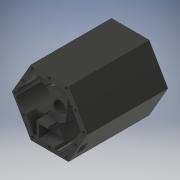
# Autodesk Inventor part: TA02
Saved by Autodesk Inventor 2017 (Build 210142000, 142)
## iProperties
Created: 2018-10-09
Part Number: TA02
Material: ABS Plastic
Document SubType Name: Modeling
Designer: Zach
Density: 1.06 g/cm^3
Appearance: Smooth - Black
Author: Zach
Autodesk Inventor part; units mm, degrees
ref_plane "YZ Plane" through (0, 0, 0) normal (1, 0, 0) x (0, 1, 0)
ref_plane "XZ Plane" through (0, 0, 0) normal (0, 1, 0) x (-1, 0, 0)
ref_plane "XY Plane" through (0, 0, 0) normal (0, 0, 1) x (1, 0, 0)
sketch "Sketch1" plane through (0, 0, 0) normal (0, 0, 1) x (1, 0, 0)
  circle A0 centre (0, 0) radius 56
  circle A1 centre (0, 0) radius 9.56
  circle A2 centre (-30, 0) radius 4
  line L0 (-39, 9) -> (-21, 9) construction
  line L1 (-21, 9) -> (-21, -9) construction
  line L2 (-21, -9) -> (-39, -9) construction
  line L3 (-39, -9) -> (-39, 9) construction
  circle A3 centre (-39, 9) radius 2
  circle A4 centre (-21, 9) radius 2
  circle A5 centre (-21, -9) radius 2
  circle A6 centre (-39, -9) radius 2
  circle A7 centre (15, 25.9808) radius 3.5
  line L4 (0, 0) -> (-30, 0) construction
  line L5 (0, 0) -> (15, 25.9808) construction
  line L6 (0, 0) -> (15, -25.9808) construction
  circle A8 centre (15, -25.9808) radius 3.5
  point P0 (-39, 0)
  point P1 (-30, 9)
  dimension "d0" = 112
  dimension "d1" = 19.12
  dimension "d2" = 8
  dimension "d3" = 30
  dimension "d4" = 18
  dimension "d5" = 18
  dimension "d6" = 4
  dimension "d7" = 4
  dimension "d8" = 4
  dimension "d9" = 4
  dimension "d10" = 7
  dimension "d11" = 30
  dimension "d12" = 120
  dimension "d13" = 30
  dimension "d14" = 7
  dimension "d15" = 120
  constraints: 14 end point, 9 centre point, 8 coincident, 2 horizontal, 2 horizontal alignment, 2 midpoint, 2 parallel, 1 perpendicular, 1 vertical alignment
  measures "d0" diameter of A0
  measures "d1" diameter of A1
  measures "d2" diameter of A2
  measures "d3" distance of L4.end point (0, 0)
  measures "d4" distance of L1.end L2.end
  measures "d5" distance of L0.end L1.end
  measures "d6" diameter of A3
  measures "d7" diameter of A4
  measures "d8" diameter of A5
  measures "d9" diameter of A6
  measures "d10" diameter of A7
  measures "d11" distance of L5.start L5.end
  measures "d12" angle of L5 L4
  measures "d13" distance of L5.start L6.end
  measures "d14" diameter of A8
  measures "d15" angle of L4 L6
extrude "Extrusion1" add sketch "Sketch1" along normal blind 5
sketch "Sketch2" plane through (0, 0, 5) normal (0, 0, 1) x (1, 0, 0)
  circle A0 centre (0, 0) radius 56 projected
  circle A1 centre (0, 0) radius 47
  dimension "d18" = 9
  constraints: 1 centre point, 1 coincident
  measures "d18" radial gap between concentric circles of A0 A1
extrude "Extrusion2" add sketch "Sketch2" along normal blind 115
sketch "Sketch3" plane through (0, 0, 5) normal (0, 0, 1) x (1, 0, 0)
  circle A0 centre (-30, 0) radius 4 projected
  circle A1 centre (0, 0) radius 9.56 projected
  circle A2 centre (15, 25.9808) radius 3.5 projected
  circle A3 centre (15, -25.9808) radius 3.5 projected
  circle A4 centre (-30, 0) radius 20
  line L0 (21.5753, 12.3695) -> (-0.0753, 24.8695)
  line L1 (-0.0753, 24.8695) -> (8.4247, 39.592)
  line L2 (8.4247, 39.592) -> (30.0753, 27.092)
  line L3 (30.0753, 27.092) -> (21.5753, 12.3695)
  line L4 (21.5753, 12.3695) -> (8.4247, 39.592) construction
  line L5 (-0.0753, 24.8695) -> (30.0753, 27.092) construction
  line L6 (0, 0) -> (-30, 0) construction
  line L7 (-0.0753, -24.8695) -> (21.5753, -12.3695)
  line L8 (21.5753, -12.3695) -> (30.0753, -27.092)
  line L9 (30.0753, -27.092) -> (8.4247, -39.592)
  line L10 (8.4247, -39.592) -> (-0.0753, -24.8695)
  circle A5 centre (0, 0) radius 47 projected
  dimension "d21" = 40
  dimension "d23" = 120
  dimension "d24" = 17
  dimension "d25" = 25
  dimension "d28" = 120
  constraints: 22 end point, 2 midpoint, 2 parallel, 1 centre point, 1 coincident, 1 horizontal, 1 perpendicular, 9 other
  measures "d21" diameter of A4
  measures "d23" angle of L6 L1
  measures "d24" distance of L0.end L1.end
  measures "d25" distance of L1.end L2.end
extrude "Extrusion3" add sketch "Sketch3" along normal blind 100 contours A4 A5 picked at (30.0502, 0)
sketch "Sketch6" plane through (-30, 0, 5) normal (0, 0, 1) x (0, 1, 0)
  circle A0 centre (0, 0) radius 4 projected
  circle A1 centre (0, 0) radius 16.5
  circle A2 centre (0, 0) radius 20 projected
  point P0 (0, -30)
  point P1 (-18.7483, -6.9642)
  dimension "d46" = 33
  constraints: 1 centre point, 1 coincident, 1 other
  measures "d46" diameter of A1
extrude "Extrusion6" add sketch "Sketch6" along normal blind 40 contours A2
sketch "Sketch14" plane through (0, 0, 0) normal (0, 0, -1) x (-1, 0, 0)
  circle A0 centre (0, 0) radius 9.56 projected
  line L0 (-56, 0) -> (-28, 48.4974)
  line L1 (-28, 48.4974) -> (28, 48.4974)
  line L2 (28, 48.4974) -> (56, 0)
  line L3 (56, 0) -> (28, -48.4974)
  line L4 (28, -48.4974) -> (-28, -48.4974)
  line L5 (-28, -48.4974) -> (-56, 0)
  circle A1 centre (0, 0) radius 56 projected
  constraints: 12 end point, 2 horizontal alignment, 1 coincident, 14 other
extrude "Extrusion12" cut sketch "Sketch14" against normal through all contours A1 L0 | L5 A1 | A1 L1 | L4 A1 | A1 L2 | L3 A1
sketch "Sketch15" plane through (0, 0, 120) normal (0, 0, 1) x (1, 0, 0)
  line L0 (-28, -48.4974) -> (28, -48.4974) projected
  line L1 (-56, 0) -> (-28, -48.4974) projected
  line L2 (-28, 48.4974) -> (-56, 0) projected
  line L3 (28, 48.4974) -> (-28, 48.4974) projected
  line L4 (56, 0) -> (28, 48.4974) projected
  line L5 (28, -48.4974) -> (56, 0) projected
  line L6 (-23.3812, -40.4974) -> (23.3812, -40.4974)
  line L7 (23.3812, -40.4974) -> (46.7624, 0)
  line L8 (46.7624, 0) -> (23.3812, 40.4974)
  line L9 (23.3812, 40.4974) -> (-23.3812, 40.4974)
  line L10 (-23.3812, 40.4974) -> (-46.7624, 0)
  line L11 (-46.7624, 0) -> (-23.3812, -40.4974)
  point P0 (0, 0)
  dimension "d80" = 8
  constraints: 12 end point, 5 other
  measures "d80" distance between parallel lines of L1 L11
extrude "Extrusion13" add sketch "Sketch15" against normal blind 15
sketch "Sketch16" plane through (0, 0, 120) normal (0, 0, 1) x (1, 0, 0)
  circle A0 centre (-51, 0) radius 2.5
  line L0 (-56, 0) -> (-28, 48.4974) projected
  circle A1 centre (-25.5, -44.1673) radius 2.5
  circle A2 centre (25.5, -44.1673) radius 2.5
  circle A3 centre (51, 0) radius 2.5
  circle A4 centre (25.5, 44.1673) radius 2.5
  circle A5 centre (-25.5, 44.1673) radius 2.5
  point P0 (0, 0)
  dimension "d83" = 5
  dimension "d90" = 5
  dimension "d93" = 360
  constraints: 6 centre point, 1 coincident, 1 horizontal alignment, 13 other
  measures "d83" diameter of A0
  measures "d90" distance of L0.start A0.centre
extrude "Extrusion14" cut sketch "Sketch16" against normal blind 50
sketch "Sketch19" plane through (-30, 0, 45) normal (0, 0, 1) x (0, -1, 0)
  circle A0 centre (0, 0) radius 20
  circle A1 centre (0, 0) radius 4 projected
  point P0 (0, 30)
  dimension "d174" = 40
  constraints: 1 centre point, 1 coincident
  measures "d174" diameter of A0
extrude "Extrusion16" cut sketch "Sketch19" along normal through all contours A0 | A1
sketch "Sketch20" plane through (0, 0, 5) normal (0, 0, 1) x (1, 0, 0)
  line L0 (8.6926, -44.0561) -> (33.8074, -29.5561)
  line L1 (33.8074, -29.5561) -> (21.3074, -7.9054)
  line L2 (21.3074, -7.9054) -> (-3.8074, -22.4054)
  line L3 (-3.8074, -22.4054) -> (8.6926, -44.0561)
  circle A0 centre (15, -25.9808) radius 3.5 projected
  line L4 (8.6926, -44.0561) -> (21.3074, -7.9054) construction
  line L5 (33.8074, -29.5561) -> (-3.8074, -22.4054) construction
  line L6 (21.5753, -12.3695) -> (30.0753, -27.092) projected
  point P0 (0, 0)
  dimension "d106" = 29
  dimension "d107" = 25
  constraints: 12 end point, 2 midpoint, 2 parallel, 2 perpendicular
  measures "d106" distance of L1.end L2.end
  measures "d107" distance of L2.end L0.start
extrude "Extrusion17" cut sketch "Sketch20" along normal through all contours L3 L2 L1 L0 | A0
sketch "Sketch21" plane through (0, 0, 0) normal (0, 0, -1) x (-1, 0, 0)
  circle A0 centre (-15, -25.9808) radius 3.5 projected
  circle A1 centre (-15, -25.9808) radius 9
  point P0 (0, 0)
  dimension "d110" = 18
  constraints: 1 centre point, 1 coincident
  measures "d110" diameter of A1
extrude "Extrusion18" cut sketch "Sketch21" against normal blind 3
sketch "Sketch22" plane through (0, 0, 5) normal (0, 0, 1) x (1, 0, 0)
  line L0 (8.6926, -44.0561) -> (33.8074, -29.5561) projected
  line L1 (33.8074, -29.5561) -> (21.3074, -7.9054) projected
  line L2 (21.3074, -7.9054) -> (-3.8074, -22.4054) projected
  line L3 (-3.8074, -22.4054) -> (8.6926, -44.0561) projected
  circle A0 centre (15, -25.9808) radius 3.5 projected
  point P0 (0, 0)
extrude "Extrusion19" add sketch "Sketch22" along normal blind 3
sketch "Sketch23" plane through (15, -25.9808, 3) normal (0, 0, -1) x (-1, 0, 0)
  circle A0 centre (0, 0) radius 3.5 projected
  circle A1 centre (0, 0) radius 9 projected
  point P0 (15, 25.9808)
extrude "Extrusion20" cut sketch "Sketch23" against normal blind 3
sketch "Sketch24" plane through (0, 0, 0) normal (0, 0, -1) x (-1, 0, 0)
  circle A0 centre (-15, 25.9808) radius 3.5 projected
  circle A1 centre (-15, 25.9808) radius 10
  point P0 (0, 0)
  dimension "d117" = 20
  constraints: 1 centre point, 1 coincident
  measures "d117" diameter of A1
extrude "Extrusion21" cut sketch "Sketch24" against normal blind 3
sketch "Sketch25" plane through (0, 0, 5) normal (0, 0, 1) x (1, 0, 0)
  line L0 (8.4247, 39.592) -> (-0.0753, 24.8695) projected
  line L1 (-0.0753, 24.8695) -> (21.5753, 12.3695) projected
  line L2 (21.5753, 12.3695) -> (30.0753, 27.092) projected
  line L3 (30.0753, 27.092) -> (8.4247, 39.592) projected
  circle A0 centre (15, 25.9808) radius 3.5 projected
  point P0 (0, 0)
extrude "Extrusion22" add sketch "Sketch25" along normal blind 6
sketch "Sketch26" plane through (15, 25.9808, 3) normal (0, 0, -1) x (-1, 0, 0)
  circle A0 centre (0, 0) radius 3.5 projected
  circle A1 centre (0, 0) radius 10 projected
  point P0 (15, -25.9808)
extrude "Extrusion23" cut sketch "Sketch26" against normal blind 2
sketch "Sketch28" plane through (0, 0, 0) normal (0, 0, -1) x (-1, 0, 0)
  circle A0 centre (39, 9) radius 2 projected
  circle A1 centre (30, 0) radius 4 projected
  circle A2 centre (39, 9) radius 4.5
  circle A3 centre (21, 9) radius 4.5
  circle A4 centre (21, -9) radius 4.5
  circle A5 centre (39, -9) radius 4.5
  point P0 (0, 0)
  dimension "d124" = 9
  dimension "d127" = 360
  constraints: 4 centre point, 1 coincident, 9 other
  measures "d124" diameter of A2
extrude "Extrusion24" cut sketch "Sketch28" against normal blind 2 contours A0 | A2 | A3 | A4 | A5
sketch "Sketch31" plane through (0, 0, 105) normal (0, 0, 1) x (1, 0, 0)
  line L0 (12.533, 28.5162) -> (7.3909, -30.2593)
  line L1 (7.3909, -30.2593) -> (29.3071, -32.1767)
  line L2 (29.3071, -32.1767) -> (34.4493, 26.5988)
  line L3 (34.4493, 26.5988) -> (12.533, 28.5162)
  line L4 (12.533, 28.5162) -> (29.3071, -32.1767) construction
  line L5 (7.3909, -30.2593) -> (34.4493, 26.5988) construction
  line L6 (9.9619, -0.8716) -> (0, 0) construction
  line L7 (0, 0) -> (0, -6.1396)
  line L8 (0, -6.1396) -> (0, -53.5118) construction
  point P0 (20.9201, -1.8303)
  dimension "d140" = 59
  dimension "d142" = 22
  dimension "d180" = 85
  dimension "d182" = 10
  constraints: 18 end point, 3 midpoint, 3 parallel, 2 vertical, 1 perpendicular
  measures "d140" distance of L1.end L2.end
  measures "d142" distance of L0.end L1.end
  measures "d180" angle of L6 L7
  measures "d182" distance of L6.start L6.end
extrude "Extrusion26" cut sketch "Sketch31" along normal blind 100 and the other way blind 55
sketch "Sketch32" plane through (0, 0, 105) normal (0, 0, 1) x (1, 0, 0)
  circle A0 centre (0, 0) radius 25
  circle A1 centre (0, 0) radius 28
  arc A2 (-0.2982, 24.9982) -> (-18.75, 16.5359) centre (0, 0) ccw
  arc A3 (-35.6931, -19.1726) -> (-35.6931, 19.1726) centre (-30, 0) ccw projected
  arc A4 (1.7022, 27.9482) -> (-21.4, 18.0566) centre (0, 0) ccw
  arc A5 (-18.75, 16.5359) -> (-21.4, 18.0566) centre (-30, 0) ccw
  line L0 (0, 25) -> (1.7022, 27.9482)
  line L1 (-0.0753, 24.8695) -> (8.4247, 39.592) projected
  point P0 (-10, 0)
  point P1 (0.8511, 26.4741)
  dimension "d146" = 3
  dimension "d147" = 50
  constraints: 13 point on circle, 5 centre point, 4 concentric, 2 coincident, 2 end point, 1 collinear, 1 midpoint, 1 point on line
  measures "d146" radial gap between concentric circles of A1 A0
  measures "d147" diameter of A0
extrude "Extrusion27" cut sketch "Sketch32" against normal blind 10 contours A0 L0 A1 A3 | A0 A3 A1 L0 | A3 A1 A0
sketch "Sketch34" plane through (0, 0, 0) normal (0, 0, -1) x (-1, 0, 0)
  circle A0 centre (-15, 25.9808) radius 3.5 projected
  circle A1 centre (-15, -25.9808) radius 3.5 projected
  circle A2 centre (-15, 25.9808) radius 5.5
  circle A3 centre (-15, -25.9808) radius 3.5 projected
  circle A4 centre (-15, -25.9808) radius 5.5
  point P0 (0, 0)
  dimension "d153" = 11
  dimension "d154" = 11
  constraints: 2 centre point, 2 coincident
  measures "d153" diameter of A2
  measures "d154" diameter of A4
extrude "Extrusion29" cut sketch "Sketch34" against normal through all contours A0 | A1 | A2 | A4
sketch "Sketch35" plane through (0, 0, 0) normal (0, 0, -1) x (-1, 0, 0)
  circle A0 centre (30, 0) radius 4 projected
  circle A1 centre (30, 0) radius 10
  line L0 (25.6411, 9) -> (34.3589, 9)
  line L1 (34.3589, -9) -> (25.6411, -9)
  line L2 (25.6411, 9) -> (25.6411, -9) construction
  line L3 (34.3589, -9) -> (34.3589, 9) construction
  circle A2 centre (30, 0) radius 16.5 construction
  circle A3 centre (21, 9) radius 2 construction
  circle A4 centre (21, 9) radius 2 projected
  point P0 (0, 0)
  dimension "d157" = 20
  dimension "d159" = 18
  constraints: 8 end point, 4 point on circle, 1 centre point, 1 coincident, 1 parallel, 1 perpendicular, 1 vertical
  measures "d157" diameter of A1
  measures "d159" distance of L1.start L0.end
extrude "Extrusion30" cut sketch "Sketch35" against normal through all contours A1 L1 L0
sketch "Sketch36" plane through (0, 0, 0) normal (0, 0, -1) x (-1, 0, 0)
  arc A0 (38.93, 4.5005) -> (34.5005, 8.93) centre (39, 9) ccw projected
  arc A1 (34.5005, -8.93) -> (38.93, -4.5005) centre (39, -9) ccw projected
  arc A2 (21.07, -4.5005) -> (25.4995, -8.93) centre (21, -9) ccw projected
  arc A3 (25.4995, 8.93) -> (21.07, 4.5005) centre (21, 9) ccw projected
  arc A4 (38.93, 4.5005) -> (34.5005, 8.93) centre (39, 9) ccw projected
  circle A5 centre (39, 9) radius 4.5
  circle A6 centre (39, -9) radius 4.5
  circle A7 centre (21, -9) radius 4.5
  arc A8 (25.4995, 8.93) -> (21.07, 4.5005) centre (21, 9) ccw projected
  circle A9 centre (21, 9) radius 4.5
  circle A10 centre (30, 0) radius 10
  arc A11 (38.93, -4.5005) -> (38.93, 4.5005) centre (30, 0) ccw projected
  arc A12 (34.5005, 8.93) -> (38.93, 4.5005) centre (39, 9) ccw
  arc A13 (25.4995, 8.93) -> (21.07, 4.5005) centre (30, 0) ccw projected
  arc A14 (25.4995, 8.93) -> (25.4995, 8.93) centre (21, 9) ccw
  arc A15 (25.4995, -8.93) -> (21.07, -4.5005) centre (21, -9) ccw
  arc A16 (38.93, -4.5005) -> (34.5005, -8.93) centre (39, -9) ccw
  line L0 (25.6411, 9) -> (34.3589, 9) projected
  line L1 (25.6411, -9) -> (34.3589, -9) projected
  arc A17 (38.93, -4.5005) -> (38.93, 4.5005) centre (30, 0) ccw
  arc A18 (21.07, 4.5005) -> (21.07, -4.5005) centre (30, 0) ccw
  arc A19 (34.5005, 8.93) -> (34.3589, 9) centre (30, 0) ccw
  arc A20 (25.6411, 9) -> (25.4995, 8.93) centre (30, 0) ccw
  arc A21 (25.4995, -8.93) -> (25.6411, -9) centre (30, 0) ccw projected
  arc A22 (25.6411, -9) -> (25.4995, -8.93) centre (30, 0) ccw
  arc A23 (34.3589, -9) -> (34.5005, -8.93) centre (30, 0) ccw
  arc A24 (21.07, 4.5005) -> (25.4995, 8.93) centre (21, 9) ccw
  arc A25 (25.6411, 9) -> (25.4995, 8.93) centre (30, 0) ccw projected
  arc A26 (25.4995, 8.93) -> (25.6411, 9) centre (30, 0) ccw
  circle A27 centre (30, 0) radius 3.5
  point P0 (0, 0)
  dimension "d164" = 7
  constraints: 22 point on circle, 12 centre point, 9 coincident, 5 concentric, 22 other
  measures "d164" diameter of A27
extrude "Extrusion31" add sketch "Sketch36" against normal blind 2 contours A10 A6 L1 A7 A9 L0 A5
sketch "Sketch40" plane through (0, 0, 105) normal (0, 0, 1) x (1, 0, 0)
  circle A0 centre (0, 0) radius 7
  circle A1 centre (0, 0) radius 9.56 projected
  dimension "d175" = 14
  constraints: 1 centre point, 1 coincident
  measures "d175" diameter of A0
extrude "Extrusion34" add sketch "Sketch40" against normal blind 92.3
sketch "Sketch41" plane through (0, 0, 105) normal (0, 0, 1) x (1, 0, 0)
  circle A0 centre (0, 0) radius 9.56 projected
extrude "Extrusion35" cut sketch "Sketch41" against normal blind 10
sketch "Sketch42" plane through (0, 0, 120) normal (0, 0, 1) x (1, 0, 0)
  circle A0 centre (-38.5359, 22.2487) radius 2.5
  line L0 (-28, 48.4974) -> (-56, 0) projected
  line L1 (-35.6931, 19.1726) -> (-23.3812, 40.4974) projected
  line L2 (-56, 0) -> (-28, 48.4974) projected
  line L3 (-42, 24.2487) -> (-38.5359, 22.2487) construction
  circle A1 centre (-38.5359, -22.2487) radius 2.5
  circle A2 centre (0, -44.4974) radius 2.5
  circle A3 centre (38.5359, -22.2487) radius 2.5
  circle A4 centre (38.5359, 22.2487) radius 2.5
  circle A5 centre (0, 44.4974) radius 2.5
  point P0 (0, 0)
  dimension "d185" = 5
  dimension "d187" = 4
  dimension "d190" = 360
  constraints: 6 centre point, 2 end point, 1 midpoint, 1 perpendicular, 13 other
  measures "d185" diameter of A0
  measures "d187" distance of L3.start L3.end
extrude "Extrusion36" cut sketch "Sketch42" against normal blind 35
sketch "Sketch43" plane through (0, 0, 0) normal (0, 0, -1) x (-1, 0, 0)
  circle A0 centre (0, 0) radius 12.7
  dimension "d194" = 25.4
  constraints: 1 centre point, 1 coincident
  measures "d194" diameter of A0
extrude "Extrusion37" cut sketch "Sketch43" against normal blind 3.2
sketch "Sketch44" plane through (0, 0, 2) normal (0, 0, 1) x (1, 0, 0)
  circle A0 centre (-30, 0) radius 3.5 projected
  arc A1 (-21.07, 4.5005) -> (-25.4995, 8.93) centre (-30, 0) ccw projected
  circle A2 centre (-30, 0) radius 10
  point P0 (0, 0)
  constraints: 1 coincident, 3 other
extrude "Extrusion38" cut sketch "Sketch44" against normal through all
sketch "Sketch45" plane through (0, 0, 105) normal (0, 0, 1) x (1, 0, 0)
  line L0 (6.638, -40.4974) -> (-23.3812, -40.4974) projected
  line L1 (-16.4115, -40.4974) -> (43.5885, -40.4974)
  line L2 (43.5885, -40.4974) -> (43.5885, -21.4974)
  line L3 (43.5885, -21.4974) -> (-16.4115, -21.4974)
  line L4 (-16.4115, -21.4974) -> (-16.4115, -40.4974)
  line L5 (28, -48.4974) -> (56, 0) projected
  line L6 (-16.4115, -21.4974) -> (-19.4115, -21.4974)
  line L7 (-19.4115, -21.4974) -> (-19.4115, -40.4974)
  line L8 (-19.4115, -40.4974) -> (-16.4115, -40.4974)
  line L9 (-16.4115, -40.4974) -> (-16.4115, -21.4974)
  line L10 (-19.4115, -21.4974) -> (-2.2346, -21.4974)
  line L11 (-2.2346, -21.4974) -> (-2.2346, -18.4974)
  line L12 (-2.2346, -18.4974) -> (-19.4115, -18.4974)
  line L13 (-19.4115, -18.4974) -> (-19.4115, -21.4974)
  line L14 (-3.8074, -22.4054) -> (8.7103, -15.1784) projected
  point P0 (0, 0)
  dimension "d199" = 19
  dimension "d203" = 3
  dimension "d204" = 3
  dimension "d213" = 60
  constraints: 24 end point, 6 parallel, 4 point on line, 3 horizontal, 3 perpendicular
  measures "d199" distance of L2.end L1.end
  measures "d203" distance of L3.end L6.end
  measures "d204" distance of L12.end L6.end
  measures "d213" distance between parallel lines of L2 L4
extrude "Extrusion39" cut sketch "Sketch45" along normal blind 10 contours L0 L4 L3 L5 L1 | L5 L2 L1
extrude "Extrusion40" add sketch "Sketch45" along normal blind 15 contours L0 L7 L6 L4 | L6 L13 L12 L11 L3
sketch "Sketch46" plane through (0, 0, 105) normal (0, 0, 1) x (1, 0, 0)
  line L0 (43.5885, -21.4974) -> (32.6188, -40.4974) projected
  line L1 (32.6188, -40.4974) -> (30.0207, -38.9974)
  line L2 (30.0207, -38.9974) -> (40.9904, -19.9974)
  line L3 (40.9904, -19.9974) -> (43.5885, -21.4974)
  line L4 (32.6188, -40.4974) -> (-12.3812, -40.4974) construction
  line L5 (-12.3812, -40.4974) -> (-12.3812, -21.4974) construction
  line L6 (-12.3812, -21.4974) -> (32.6188, -21.4974) construction
  line L7 (32.6188, -21.4974) -> (32.6188, -40.4974) construction
  line L8 (32.6188, -36.9974) -> (41.5677, -36.9974) construction
  line L9 (41.5677, -36.9974) -> (41.5677, -24.9974) construction
  line L10 (41.5677, -24.9974) -> (32.6188, -24.9974) construction
  line L11 (32.6188, -24.9974) -> (32.6188, -36.9974)
  line L12 (43.5885, -21.4974) -> (41.5677, -24.9974)
  line L13 (56, 0) -> (28, -48.4974) projected
  line L14 (41.5677, -24.9974) -> (38.1036, -24.9974)
  line L15 (38.1036, -24.9974) -> (40.9904, -19.9974)
  line L16 (43.5885, -21.4974) -> (40.9904, -19.9974)
  line L17 (32.6188, -40.4974) -> (34.6395, -36.9974)
  line L18 (34.6395, -36.9974) -> (32.6188, -36.9974)
  line L19 (32.6188, -36.9974) -> (31.1754, -36.9974)
  line L20 (31.1754, -36.9974) -> (31.1754, -39.6641)
  line L21 (31.1754, -39.6641) -> (32.6188, -40.4974)
  circle A0 centre (38.5359, -22.2487) radius 2.5 projected
  circle A1 centre (38.5359, -22.2487) radius 2.5 projected
  arc A2 (38.2563, -24.733) -> (40.5476, -20.7644) centre (38.5359, -22.2487) ccw
  line L22 (40.9904, -19.9974) -> (40.5476, -20.7644)
  line L23 (38.2563, -24.733) -> (38.1036, -24.9974)
  line L24 (31.1754, -39.6641) -> (31.1754, -42.9974)
  line L25 (32.6188, -40.4974) -> (31.1754, -42.9974)
  line L26 (32.6188, -21.4974) -> (32.6188, -24.9974)
  line L27 (38.1036, -24.9974) -> (32.6188, -24.9974)
  line L28 (32.6188, -21.4974) -> (36.1515, -21.4974)
  arc A3 (36.1515, -21.4974) -> (38.2563, -24.733) centre (38.5359, -22.2487) ccw
  point P0 (0, 0)
  point P1 (32.6188, -30.9974)
  dimension "d207" = 3
  dimension "d208" = 45
  dimension "d209" = 19
  dimension "d210" = 12
  constraints: 54 end point, 11 point on line, 10 point on circle, 7 perpendicular, 6 collinear, 5 parallel, 4 horizontal, 2 centre point, 2 midpoint, 2 vertical, 1 coincident, 1 concentric
  measures "d207" distance of L0.end L1.end
  measures "d208" distance of L5.end L6.end
  measures "d209" distance of L4.end L5.end
  measures "d210" distance of L8.end L9.end
extrude "Extrusion41" add sketch "Sketch46" along normal blind 15 contours L0 L14 L2 A0 L3 | L0 L1 L20 L19 L18 | L27 L26 L28 A0 L2 | L13 L24 L1
equation "\"d3\" = d11"
equation "\"d13\" = d11"
body "Solid1"
